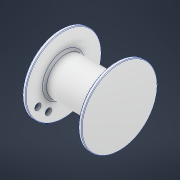
# Autodesk Inventor part: secureingReel
Saved by Autodesk Inventor 2021 (Build 250183000, 183)
## iProperties
Created: 2021-06-22
Part Number: secureingReel
Material: Aluminum 6061
Document SubType Name: Modeling
Designer: Watchdog
Density: 2.7 g/cm^3
Appearance: Aluminum - Flat
Author: Watchdog
Autodesk Inventor part; units mm, degrees
ref_plane "YZ Plane" through (0, 0, 0) normal (1, 0, 0) x (0, 1, 0)
ref_plane "XZ Plane" through (0, 0, 0) normal (0, 1, 0) x (-1, 0, 0)
ref_plane "XY Plane" through (0, 0, 0) normal (0, 0, 1) x (1, 0, 0)
sketch "Sketch1" plane through (0, 0, 0) normal (0, 0, 1) x (1, 0, 0)
  line L0 (-28, 36) -> (-25, 36)
  line L1 (-25, 36) -> (-25, 18)
  line L2 (-25, 18) -> (0, 18)
  line L3 (0, 18) -> (0, 0)
  line L4 (0, 0) -> (-28, 0)
  line L5 (-28, 0) -> (-28, 36)
  line L6 (0, 17.0507) -> (0, -8.2074)
  line L7 (28, 36) -> (25, 36)
  line L8 (25, 36) -> (25, 18)
  line L9 (25, 18) -> (0, 18)
  line L10 (0, 0) -> (28, 0)
  line L11 (28, 0) -> (28, 36)
  dimension "d0" = 3
  dimension "d1" = 18
  dimension "d2" = 36
  dimension "d3" = 25
  constraints: 24 end point, 4 perpendicular, 4 symmetric about line, 2 vertical, 1 horizontal, 1 point on line
  measures "d0" distance between parallel lines of L1 L5
  measures "d1" distance between parallel lines of L4 L2
  measures "d2" distance between parallel lines of L4 L0
  measures "d3" distance from line of L3.end L1
revolve "Revolution1" add sketch "Sketch1" angle 360 about axis through (0, 0, 0) along (1, 0, 0)
sketch "Sketch2" plane through (-25, 0, 0) normal (1, 0, 0) x (0, 0, -1)
  circle A0 centre (0, 0) radius 18 projected
  point P0 (-24.3609, -14.1125)
  point P1 (-14.4451, -23.0443)
hole "Hole1" at (-25, -14.1125, 24.3609) at (-25, -23.0443, 14.4451) direction (-1, 0, 0) diameter 6 depth 3 tip angle 118
sketch "Sketch3" plane through (-28, 0, 0) normal (-1, 0, 0) x (0, 0, 1)
  circle A0 centre (0, 0) radius 3.5
  line L0 (3.1623, 1.5) -> (4.4623, 1.5)
  line L1 (4.4623, 1.5) -> (4.4623, -1.5)
  line L2 (4.4623, -1.5) -> (3.1623, -1.5)
  line L3 (3.1623, -1.5) -> (3.1623, 1.5)
  dimension "d12" = 7
  dimension "d13" = 3
  dimension "d14" = 1.3
  constraints: 8 end point, 2 parallel, 2 point on circle, 1 centre point, 1 coincident, 1 horizontal, 1 perpendicular
  measures "d12" diameter of A0
  measures "d13" distance between parallel lines of L2 L0
  measures "d14" distance between parallel lines of L3 L1
extrude "Extrusion1" cut sketch "Sketch3" against normal blind 22
chamfer "Chamfer1" distance 0.5 angle 45 4 edges at (-28, 0, -3.5) (-28, 1.5, 3.8123) (-28, 0, 4.4623) (-28, -1.5, 3.8123)
fillet "Fillet1" radius 2 2 edges at (-25, -18, 0) (25, -18, 0)
fillet "Fillet2" radius 0.5 4 edges at (-28, -36, 0) (-25, -36, 0) (25, -36, 0) (28, -36, 0)
equation "\"d0\" = tedge"
equation "\"d1\" = r1"
equation "\"d2\" = r2"
equation "\"d3\" = 0.5 * win"
equation "\"tedge\" = 3"
equation "\"r1\" = 18"
equation "\"r2\" = 36"
equation "\"win\" = 50"
body "Solid1"
